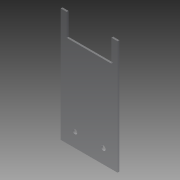
# Autodesk Inventor part: Servo Mount
Saved by Autodesk Inventor 2014 (Build 180170000, 170)
## iProperties
Created: 2014-02-24
Part Number: Servo Mount
Material: Polycarbonate, Clear
Document SubType Name: Modeling
Designer: Andrew Toennies
Mass: 8.25658 g
Surface Area: 92.572 cm^2
Volume: 6.88048 cm^3
Density: 1.2 g/cm^3
Appearance: Polycarbonate - Clear
Author: Andrew Toennies
Autodesk Inventor part; units mm, degrees
ref_plane "YZ Plane" through (0, 0, 0) normal (1, 0, 0) x (0, 1, 0)
ref_plane "XZ Plane" through (0, 0, 0) normal (0, 1, 0) x (-1, 0, 0)
ref_plane "XY Plane" through (0, 0, 0) normal (0, 0, 1) x (1, 0, 0)
sketch "Sketch1" plane through (0, 0, 0) normal (0, 0, 1) x (1, 0, 0)
  line L0 (0, 0) -> (50.8, 0)
  line L1 (50.8, 0) -> (50.8, 101.6)
  line L2 (0, 0) -> (0, 101.6)
  line L3 (0, 101.6) -> (5.461, 101.6)
  line L4 (5.461, 101.6) -> (5.461, 81.534)
  line L5 (5.461, 81.534) -> (45.339, 81.534)
  line L6 (45.339, 81.534) -> (45.339, 101.6)
  line L7 (45.339, 101.6) -> (50.8, 101.6)
  circle A0 centre (12.7, 12.7) radius 2.0701
  circle A1 centre (38.1, 12.7) radius 2.0701
  dimension "d0" = 50.8
  dimension "d1" = 101.6
  dimension "d2" = 101.6
  dimension "d3" = 5.461
  dimension "d4" = 20.066
  dimension "d5" = 5.461
  dimension "d6" = 4.1402
  dimension "d7" = 4.1402
  dimension "d8" = 12.7
  dimension "d9" = 12.7
  dimension "d10" = 12.7
  dimension "d11" = 12.7
  constraints: 16 end point, 3 parallel, 3 perpendicular, 2 centre point, 1 collinear, 1 horizontal
  measures "d0" distance of L0.start L0.end
  measures "d1" distance of L0.end L1.end
  measures "d2" distance of L0.start L2.end
  measures "d3" distance of L2.end L3.end
  measures "d4" distance of L3.end L4.end
  measures "d5" distance between parallel lines of L6 L1
  measures "d6" diameter of A0
  measures "d7" diameter of A1
  measures "d8" distance from line of L1 A1.centre
  measures "d9" distance from line of L0 A1.centre
  measures "d10" distance from line of L0 A0.centre
  measures "d11" distance from line of L2 A0.centre
extrude "Extrusion1" add sketch "Sketch1" along normal blind 1.5875
body "Solid1"
